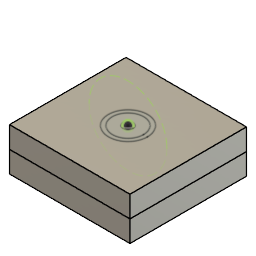
Spur Gear v5 (Autodesk Fusion 360 design; units mm, degrees)
description: Spur Gear; Module: 2.0; Num Teeth: 20; Pressure Angle: 20.0; Backlash: 0.30 mm
Autodesk Fusion 360 part; units mm, degrees
note: some values were not read from the file. Chosen so that the rebuilt part matches the saved one: which bodies a step acts on; which face or edge a step refers to.
sketch "Sketch1" plane through (0, 0, 0) normal (0, 1, 0) x (1, 0, 0)
  circle A0 centre (0, 0) radius 10
  circle A1 centre (0, 0) radius 8
  circle A2 centre (0, 0) radius 2.5
  dimension "d1" = 20
  dimension "d2" = 16
  dimension "d3" = 5
  constraint coincident A0.centre A1.centre
  measures "d1" diameter of A0
  measures "d2" diameter of A1
  measures "d3" diameter of A2
sketch "Sketch1 (2)" plane through (0, 0, 0) normal (0, 0, 1) x (1, 0, 0) in component "Spur Gear (20 teeth)"
  circle A0 centre (0, 0) radius 17.5492
  circle A1 centre (0, 0) radius 5
extrude "Extrude1" add sketch "Sketch1 (2)" along normal blind 10 makes body 1 in component "Spur Gear (20 teeth)"
sketch "Sketch2" plane through (0, 0, 0) normal (0, 0, 1) x (1, 0, 0) in component "Spur Gear (20 teeth)"
  spline S0 degree 5 poles (18.7183, -1.6834) (18.7277, -1.6843) (18.7465, -1.6857) (18.7747, -1.6871) (18.8123, -1.6876) (18.8595, -1.6862) (18.9066, -1.6834) (18.9539, -1.6797) (19.0011, -1.6756) (19.0484, -1.6712) (19.0957, -1.6664) (19.143, -1.6611) (19.1904, -1.6553) (19.2377, -1.6488) (19.285, -1.6417) (19.3324, -1.6338) (19.3797, -1.6255) (19.427, -1.6167) (19.4744, -1.6075) (19.5217, -1.5979) (19.569, -1.5879) (19.6163, -1.5776) (19.6636, -1.5668) (19.7109, -1.5556) (19.7582, -1.544) (19.8054, -1.532) (19.8527, -1.5195) (19.8999, -1.5068) (19.9471, -1.4936) (19.9943, -1.4801) (20.0414, -1.4663) (20.0886, -1.4521) (20.1357, -1.4376) (20.1828, -1.4228) (20.2299, -1.4076) (20.2769, -1.392) (20.3239, -1.3762) (20.3709, -1.36) (20.4179, -1.3435) (20.4648, -1.3267) (20.5117, -1.3096) (20.5586, -1.2921) (20.6054, -1.2744) (20.6522, -1.2564) (20.699, -1.238) (20.7457, -1.2194) (20.7924, -1.2005) (20.8391, -1.1812) (20.8857, -1.1617) (20.9323, -1.1419) (20.9789, -1.1219) (21.0254, -1.1015) (21.0718, -1.0809) (21.1183, -1.0599) (21.1646, -1.0388) (21.211, -1.0173) (21.2573, -0.9956) (21.3035, -0.9736) (21.3497, -0.9513) (21.3959, -0.9288) (21.442, -0.906) (21.4881, -0.8829) (21.5341, -0.8596) (21.5801, -0.836) (21.626, -0.8121) (21.6719, -0.7881) (21.7177, -0.7637) (21.7634, -0.7391) (21.8092, -0.7143) (21.8548, -0.6892) (21.9004, -0.6638) (21.9369, -0.6433) (21.9642, -0.6279) (21.9824, -0.6175) (21.9915, -0.6123) knots 0 0 0 0 0 0 0.01428571 0.02857143 0.04285714 0.05714286 0.07142857 0.08571429 0.1 0.11428571 0.12857143 0.14285714 0.15714286 0.17142857 0.18571429 0.2 0.21428571 0.22857143 0.24285714 0.25714286 0.27142857 0.28571429 0.3 0.31428571 0.32857143 0.34285714 0.35714286 0.37142857 0.38571429 0.4 0.41428571 0.42857143 0.44285714 0.45714286 0.47142857 0.48571429 0.5 0.51428571 0.52857143 0.54285714 0.55714286 0.57142857 0.58571429 0.6 0.61428571 0.62857143 0.64285714 0.65714286 0.67142857 0.68571429 0.7 0.71428571 0.72857143 0.74285714 0.75714286 0.77142857 0.78571429 0.8 0.81428571 0.82857143 0.84285714 0.85714286 0.87142857 0.88571429 0.9 0.91428571 0.92857143 0.94285714 0.95714286 0.97142857 0.98571429 1 1 1 1 1 1
  spline S1 degree 5 poles (18.7183, 1.6834) (18.7277, 1.6843) (18.7465, 1.6857) (18.7747, 1.6871) (18.8123, 1.6876) (18.8595, 1.6862) (18.9066, 1.6834) (18.9539, 1.6797) (19.0011, 1.6756) (19.0484, 1.6712) (19.0957, 1.6664) (19.143, 1.6611) (19.1904, 1.6553) (19.2377, 1.6488) (19.285, 1.6417) (19.3324, 1.6338) (19.3797, 1.6255) (19.427, 1.6167) (19.4744, 1.6075) (19.5217, 1.5979) (19.569, 1.5879) (19.6163, 1.5776) (19.6636, 1.5668) (19.7109, 1.5556) (19.7582, 1.544) (19.8054, 1.532) (19.8527, 1.5195) (19.8999, 1.5068) (19.9471, 1.4936) (19.9943, 1.4801) (20.0414, 1.4663) (20.0886, 1.4521) (20.1357, 1.4376) (20.1828, 1.4228) (20.2299, 1.4076) (20.2769, 1.392) (20.3239, 1.3762) (20.3709, 1.36) (20.4179, 1.3435) (20.4648, 1.3267) (20.5117, 1.3096) (20.5586, 1.2921) (20.6054, 1.2744) (20.6522, 1.2564) (20.699, 1.238) (20.7457, 1.2194) (20.7924, 1.2005) (20.8391, 1.1812) (20.8857, 1.1617) (20.9323, 1.1419) (20.9789, 1.1219) (21.0254, 1.1015) (21.0718, 1.0809) (21.1183, 1.0599) (21.1646, 1.0388) (21.211, 1.0173) (21.2573, 0.9956) (21.3035, 0.9736) (21.3497, 0.9513) (21.3959, 0.9288) (21.442, 0.906) (21.4881, 0.8829) (21.5341, 0.8596) (21.5801, 0.836) (21.626, 0.8121) (21.6719, 0.7881) (21.7177, 0.7637) (21.7634, 0.7391) (21.8092, 0.7143) (21.8548, 0.6892) (21.9004, 0.6638) (21.9369, 0.6433) (21.9642, 0.6279) (21.9824, 0.6175) (21.9915, 0.6123) knots 0 0 0 0 0 0 0.01428571 0.02857143 0.04285714 0.05714286 0.07142857 0.08571429 0.1 0.11428571 0.12857143 0.14285714 0.15714286 0.17142857 0.18571429 0.2 0.21428571 0.22857143 0.24285714 0.25714286 0.27142857 0.28571429 0.3 0.31428571 0.32857143 0.34285714 0.35714286 0.37142857 0.38571429 0.4 0.41428571 0.42857143 0.44285714 0.45714286 0.47142857 0.48571429 0.5 0.51428571 0.52857143 0.54285714 0.55714286 0.57142857 0.58571429 0.6 0.61428571 0.62857143 0.64285714 0.65714286 0.67142857 0.68571429 0.7 0.71428571 0.72857143 0.74285714 0.75714286 0.77142857 0.78571429 0.8 0.81428571 0.82857143 0.84285714 0.85714286 0.87142857 0.88571429 0.9 0.91428571 0.92857143 0.94285714 0.95714286 0.97142857 0.98571429 1 1 1 1 1 1
  arc A0 (21.9915, -0.6123) -> (21.9915, 0.6123) centre (0, 0) ccw
  line L0 (17.4687, -1.572) -> (18.7183, -1.6834)
  line L1 (17.4687, 1.572) -> (18.7183, 1.6834)
  line L2 (17.4687, -1.572) -> (17.4687, 1.572)
  point P0 (18.9485, -1.6801)
  point P1 (19.1805, -1.6564)
  point P2 (19.4135, -1.6191)
  point P3 (19.6472, -1.5705)
  point P4 (19.8815, -1.5117)
  point P5 (20.1162, -1.4436)
  point P6 (20.3511, -1.3668)
  point P7 (20.5861, -1.2817)
  point P8 (20.821, -1.1886)
  point P9 (21.0559, -1.0879)
  point P10 (21.2904, -0.9797)
  point P11 (21.5246, -0.8643)
  point P12 (21.7583, -0.7418)
  point P13 (18.9485, 1.6801)
  point P14 (19.1805, 1.6564)
  point P15 (19.4135, 1.6191)
  point P16 (19.6472, 1.5705)
  point P17 (19.8815, 1.5117)
  point P18 (20.1162, 1.4436)
  point P19 (20.3511, 1.3668)
  point P20 (20.5861, 1.2817)
  point P21 (20.821, 1.1886)
  point P22 (21.0559, 1.0879)
  point P23 (21.2904, 0.9797)
  point P24 (21.5246, 0.8643)
  point P25 (21.7583, 0.7418)
extrude "Extrude2" add sketch "Sketch2" along normal blind 10 bodies 1 in component "Spur Gear (20 teeth)"
fillet "Fillet1" radius 0.5 2 edges at (17.4786, -1.5728, 5) (17.4786, 1.5728, 5) on bodies 1 in component "Spur Gear (20 teeth)"
pattern_circular "C-Pattern1" count 20 over 360 about axis through (0, 0, 0) along (0, 0, 1) of "Extrude2", "Fillet1" in component "Spur Gear (20 teeth)"
sketch "Sketch3" plane through (0, 0, 0) normal (0, 0, 1) x (1, 0, 0) in component "Spur Gear (20 teeth)"
  circle A0 centre (0, 0) radius 20 construction
ref_plane "WorkPlane1" through (0, 0, 5) normal (0, 0, 1) x (1, 0, 0)
sketch "Sketch2 (2)" plane through (0, 0, 5) normal (0, 0, 1) x (1, 0, 0)
  line L0 (31, -30) -> (-31, -30)
  line L1 (-31, -30) -> (-31, 30)
  line L2 (-31, 30) -> (31, 30)
  line L3 (31, 30) -> (31, -30)
  line L4 (31, -30) -> (-31, 30) construction
  line L5 (-31, -30) -> (31, 30) construction
  constraint horizontal L0
  constraint perpendicular L0 L1
  constraint parallel L0 L2
  constraint parallel L1 L3
  constraint coincident L4 origin
  constraint coincident L5 origin
extrude "Extrude1'" add sketch "Sketch2 (2)" along normal blind 11 and the other way blind 11 separate body makes body 2
combine "Combine1" operation cut target body 2 tool bodies 1 keep tools result as body 3 in component "Mold Top"
ref_plane "WorkPlane2" through (0, 0, 5) normal (0, 0, 1) x (1, 0, 0)
split "Split1" by plane through (0, 0, 5) normal (0, 0, 1) bodies 3 makes body 4 at (-10.3333, -10, 16) in component "Mold Top"
sphere "SpherePrimitive1" add diameter 8 placed x (1, 0, 0) y (0, 1, 0) z (0, 0, 1) at (24, -25, 5) bodies 3 in component "Mold Top"
pattern_linear "R-Pattern1" count 2 spacing 50 along (0, 1, 0) count 2 spacing 50 along (-1, 0, 0) of 1 faces at (20.0874, -25, 5.8316) on bodies 3 in component "Mold Top"
combine "Combine1'" operation cut target body 4 tool bodies 3 keep tools result as body 5 in component "Mold Bottom"
delete_body "RemoveBody1" bodies 4 in component "Mold Top"
hole "Hole1" at (-11.3988, 6.2047, -6) direction (0, 0, 1) diameter 5 depth 7 tip angle 180 bodies 3 in component "Mold Top"
component "Spur Gear (20 teeth)" placed x (1, 0, 0) y (0, 1, 0) z (0, 0, 1) at (0, 0, 0)
component "Mold Top" placed x (1, 0, 0) y (0, 0, -1) z (0, 1, 0) at (0, -16, 0)
component "Mold Bottom" placed x (1, 0, 0) y (0, 0, -1) z (0, 1, 0) at (0, -16, 0)
hidden bodies 1
named bodies: "Mold Top", "Mold Bottom"
